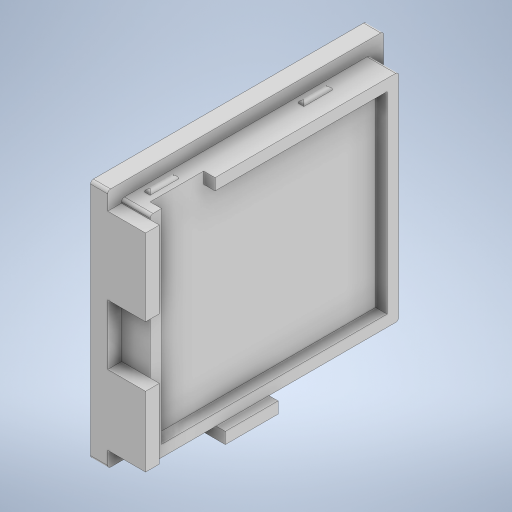
# Autodesk Inventor part: Enclosure_Bottom
Saved by Autodesk Inventor 2023 (Build 270158030, 158C)
## iProperties
Created: 2023-07-27
Part Number: Enclosure_Bottom
Material: Generic
Document SubType Name: Modeling
Designer: Tropaion
Density: 1 g/cm^3
Appearance: Default
Author: Tropaion
Autodesk Inventor part; units mm, degrees
ref_plane "YZ Plane" through (0, 0, 0) normal (1, 0, 0) x (0, 1, 0)
ref_plane "XZ Plane" through (0, 0, 0) normal (0, 1, 0) x (-1, 0, 0)
ref_plane "XY Plane" through (0, 0, 0) normal (0, 0, 1) x (1, 0, 0)
sketch "Sketch1" plane through (0, 0, 0) normal (1, 0, 0) x (0, 1, 0)
  line L0 (9.8886, 10.374) -> (-32.1114, 10.374)
  line L1 (-32.1114, 10.374) -> (-32.1114, -37.736)
  line L2 (-32.1114, -37.736) -> (9.8886, -37.736)
  line L3 (9.8886, -37.736) -> (9.8886, 10.374)
  point P0 (0, 0)
  dimension "d0" = 42
  dimension "d1" = 48.11
  constraints: 8 end point, 2 parallel, 1 horizontal, 1 perpendicular
  measures "d0" distance of L2.end L1.end
  measures "d1" distance of L1.end L0.end
extrude "Extrusion1" add sketch "Sketch1" along normal blind 3
sketch "Sketch2" plane through (3, 0, 0) normal (1, 0, 0) x (0, 0, -1)
  line L0 (-7.974, 7.4886) -> (35.336, 7.4886)
  line L1 (35.336, 7.4886) -> (35.336, -30.1114)
  line L2 (35.336, -30.1114) -> (-7.974, -30.1114)
  line L3 (-7.974, -30.1114) -> (-7.974, 7.4886)
  line L4 (37.736, 9.8886) -> (-10.374, 9.8886) projected
  line L5 (-10.374, 9.8886) -> (-10.374, -32.1114) projected
  line L6 (-10.374, -32.1114) -> (37.736, -32.1114) projected
  point P0 (0, 0)
  dimension "d4" = 43.31
  dimension "d6" = 2.4
  dimension "d7" = 2.4
  dimension "d20" = 2
  constraints: 8 end point, 2 parallel, 1 horizontal, 1 perpendicular
  measures "d4" distance of L1.end L2.end
  measures "d6" distance between parallel lines of L4 L0
  measures "d7" distance between parallel lines of L5 L3
  measures "d20" distance between parallel lines of L6 L2
extrude "Extrusion2" add sketch "Sketch2" along normal blind 3
fillet "Fillet1" radius 0.5 4 edges at (1.5, 9.8886, 10.374) (1.5, 9.8886, -37.736) (1.5, -32.1114, 10.374) (1.5, -32.1114, -37.736)
sketch "Sketch3" plane through (3, 0, 0) normal (1, 0, 0) x (0, 0, -1)
  line L0 (-10.374, 9.3886) -> (-10.374, -31.6114) projected
  line L1 (-7.974, -30.1114) -> (-7.974, 7.4886) projected
  line L2 (-10.374, -29.3114) -> (-7.974, -29.3114)
  line L3 (-7.974, -29.3114) -> (-7.974, -17.1114)
  line L4 (-7.974, -17.1114) -> (-10.374, -17.1114)
  line L5 (-10.374, -17.1114) -> (-10.374, -29.3114)
  line L6 (-9.874, -32.1114) -> (37.236, -32.1114) projected
  point P0 (0, 0)
  point P1 (-7.974, -29.6114)
  point P2 (-7.974, 6.9886)
  point P3 (-7.974, -29.3114)
  dimension "d12" = 12.2
  dimension "d13" = 2.8
  constraints: 8 end point, 2 parallel, 2 point on line, 1 horizontal, 1 perpendicular
  measures "d12" distance of L3.end L2.end
  measures "d13" distance between parallel lines of L2 L6
extrude "PowerSocket" add sketch "Sketch3" along normal blind 6.6
sketch "Sketch5" plane through (3, 0, 0) normal (1, 0, 0) x (0, 0, -1)
  line L0 (-10.374, 9.3886) -> (-10.374, -17.1114) projected
  line L1 (-7.974, -17.1114) -> (-7.974, 7.4886) projected
  line L2 (-10.374, -6.6114) -> (-7.974, -6.6114)
  line L3 (-7.974, -6.6114) -> (-7.974, 6.7886)
  line L4 (-7.974, 6.7886) -> (-10.374, 6.7886)
  line L5 (-10.374, 6.7886) -> (-10.374, -6.6114)
  line L6 (-7.974, -17.1114) -> (-10.374, -17.1114) projected
  line L7 (35.336, 7.4886) -> (-7.974, 7.4886) projected
  line L8 (37.236, 9.8886) -> (-9.874, 9.8886) projected
  point P0 (0, 0)
  point P1 (-10.374, 6.7886)
  point P2 (-7.974, -6.6114)
  dimension "d21" = 13.4
  dimension "d75" = 3.1
  constraints: 8 end point, 2 parallel, 2 point on line, 1 horizontal, 1 perpendicular
  measures "d21" distance of L3.end L2.end
  measures "d75" distance between parallel lines of L4 L8
extrude "RJ-12" add sketch "Sketch5" along normal blind 6.6 contours L4 L1 L2 L0
sketch "Sketch6" plane through (3, 0, 0) normal (1, 0, 0) x (0, 0, -1)
  line L0 (-9.874, -32.1114) -> (37.236, -32.1114) projected
  line L1 (-7.974, -30.1114) -> (35.336, -30.1114) projected
  line L2 (12.726, -32.1114) -> (3.526, -32.1114)
  line L3 (3.526, -32.1114) -> (3.526, -30.1114)
  line L4 (3.526, -30.1114) -> (12.726, -30.1114)
  line L5 (12.726, -30.1114) -> (12.726, -32.1114)
  line L6 (-10.374, -29.3114) -> (-10.374, -31.6114) projected
  point P0 (0, 0)
  dimension "d25" = 9.2
  dimension "d26" = 13.9
  constraints: 8 end point, 2 parallel, 2 point on line, 1 horizontal, 1 perpendicular
  measures "d25" distance of L3.end L4.end
  measures "d26" distance between parallel lines of L6 L3
extrude "USB-C" add sketch "Sketch6" along normal blind 6.6
sketch "Sketch7" plane through (6, 0, 0) normal (1, 0, 0) x (0, 0, -1)
  line L0 (35.336, 7.4886) -> (-7.974, 7.4886) projected
  line L1 (-7.974, 7.4886) -> (-5.974, 7.4886)
  line L2 (-5.974, 7.4886) -> (-5.974, -30.1114)
  line L3 (-7.974, -30.1114) -> (3.526, -30.1114) projected
  line L4 (-5.974, -30.1114) -> (-7.974, -30.1114)
  line L5 (-10.374, -29.3114) -> (-10.374, -31.6114) projected
  line L6 (-7.974, 7.4886) -> (-7.974, -17.1114) projected
  line L7 (-7.974, -30.1114) -> (-7.974, 7.4886)
  line L8 (35.336, -30.1114) -> (12.726, -30.1114) projected
  line L9 (-5.974, -30.1114) -> (35.336, -30.1114)
  line L10 (35.336, -30.1114) -> (35.336, -28.1114)
  line L11 (35.336, 7.4886) -> (35.336, -30.1114) projected
  line L12 (35.336, -28.1114) -> (-5.974, -28.1114)
  line L13 (35.336, -28.1114) -> (35.336, 7.4886)
  line L14 (35.336, 7.4886) -> (33.336, 7.4886)
  line L15 (33.336, 7.4886) -> (33.336, -28.1114)
  line L16 (33.336, 7.4886) -> (3.336, 7.4886)
  line L17 (3.336, 7.4886) -> (3.336, 5.4886)
  line L18 (3.336, 5.4886) -> (33.336, 5.4886)
  point P0 (0, 0)
  point P1 (-7.974, 6.7886)
  point P2 (-7.974, 6.6886)
  dimension "d29" = 2
  dimension "d30" = 2
  dimension "d31" = 2
  dimension "d32" = 2
  dimension "d33" = 30
  dimension "d34" = 2
  constraints: 26 end point, 8 point on line, 7 perpendicular, 1 collinear
  measures "d29" distance of L0.end L1.end
  measures "d30" distance of L2.end L4.end
  measures "d31" distance of L8.start L10.end
  measures "d32" distance of L0.start L14.end
  measures "d33" distance of L14.end L16.end
  measures "d34" distance of L16.end L17.end
extrude "Extrusion7" add sketch "Sketch7" along normal blind 2 contours L11 L12 L15 L0 | L15 L18 L17 L0 | L10 L8 L9 L3 L2 L12 | L2 L3 L7 L6 L0
sketch "Sketch8" plane through (3, -30.1114, -3.526) normal (0, -1, 0) x (1, 0, 0)
  line L0 (2, 8.5) -> (1, 8.5)
  line L1 (1, 8.5) -> (1, 3.5)
  line L2 (1, 3.5) -> (2, 3.5)
  line L3 (2, 3.5) -> (2, 8.5)
  line L4 (0, 11.5) -> (5, 11.5) projected
  line L5 (5, 11.5) -> (5, 0) projected
  line L6 (0, 13.4) -> (0, 0) projected
  point P0 (-3, 3.526)
  point P1 (2, 6)
  dimension "d37" = 1
  dimension "d38" = 5
  dimension "d39" = 5.5
  dimension "d60" = 1
  constraints: 8 end point, 2 parallel, 1 horizontal, 1 midpoint, 1 perpendicular
  measures "d37" distance of L2.end L1.end
  measures "d38" distance of L1.end L0.end
  measures "d39" distance from line of L4 point (2, 6)
  measures "d60" distance between parallel lines of L6 L1
extrude "Extrusion8" add sketch "Sketch8" along normal blind 0.5
fillet "Fillet3" radius 0.5 4 edges at (5, -30.6114, 2.474) (4, -30.6114, 2.474) (4.5, -30.6114, 4.974) (4.5, -30.6114, -0.026)
sketch "Sketch9" plane through (3, -30.1114, -35.336) normal (0, -1, 0) x (1, 0, 0)
  line L0 (2, 13.5) -> (1, 13.5)
  line L1 (1, 13.5) -> (1, 8.5)
  line L2 (1, 8.5) -> (2, 8.5)
  line L3 (2, 8.5) -> (2, 13.5)
  line L4 (5, 22.61) -> (5, 0) projected
  line L5 (0, 0) -> (5, 0) projected
  line L6 (0, 22.61) -> (0, -1.9) projected
  point P0 (-3, 35.336)
  point P1 (2, 11)
  dimension "d44" = 1
  dimension "d45" = 5
  dimension "d47" = 11
  dimension "d59" = 1
  constraints: 8 end point, 2 parallel, 1 horizontal, 1 midpoint, 1 perpendicular
  measures "d44" distance of L2.end L1.end
  measures "d45" distance of L1.end L0.end
  measures "d47" distance from line of L5 point (2, 11)
  measures "d59" distance between parallel lines of L6 L1
extrude "Extrusion9" add sketch "Sketch9" along normal blind 0.5
fillet "Fillet4" radius 0.5 4 edges at (5, -30.6114, -24.336) (4, -30.6114, -24.336) (4.5, -30.6114, -21.836) (4.5, -30.6114, -26.836)
sketch "Sketch10" plane through (3, 7.4886, 7.974) normal (0, 1, 0) x (1, 0, 0)
  line L0 (2, 34.81) -> (1, 34.81)
  line L1 (1, 34.81) -> (1, 29.81)
  line L2 (1, 29.81) -> (2, 29.81)
  line L3 (2, 29.81) -> (2, 34.81)
  line L4 (5, 43.31) -> (5, 11.31) projected
  line L5 (0, 43.31) -> (5, 43.31) projected
  line L6 (0, 45.21) -> (0, -1.9) projected
  point P0 (-3, 7.974)
  point P1 (2, 32.31)
  dimension "d51" = 1
  dimension "d52" = 5
  dimension "d54" = 11
  dimension "d58" = 1
  constraints: 8 end point, 2 parallel, 1 horizontal, 1 midpoint, 1 perpendicular
  measures "d51" distance of L2.end L1.end
  measures "d52" distance of L1.end L0.end
  measures "d54" distance from line of L5 point (2, 32.31)
  measures "d58" distance between parallel lines of L6 L1
extrude "Extrusion10" add sketch "Sketch10" along normal blind 0.5
fillet "Fillet5" radius 0.5 4 edges at (5, 7.9886, -24.336) (4, 7.9886, -24.336) (4.5, 7.9886, -26.836) (4.5, 7.9886, -21.836)
sketch "Sketch11" plane through (3, 7.4886, 7.974) normal (0, 1, 0) x (1, 0, 0)
  line L0 (2, 8) -> (1, 8)
  line L1 (1, 8) -> (1, 3)
  line L2 (1, 3) -> (2, 3)
  line L3 (2, 3) -> (2, 8)
  line L4 (0, 45.21) -> (0, -1.9) projected
  line L5 (0, 0) -> (5, 0) projected
  point P0 (-3, 7.974)
  point P1 (1, 5.5)
  dimension "d61" = 1
  dimension "d62" = 5
  dimension "d63" = 1
  dimension "d64" = 5.5
  constraints: 8 end point, 2 parallel, 1 horizontal, 1 midpoint, 1 perpendicular
  measures "d61" distance of L2.end L1.end
  measures "d62" distance of L1.end L0.end
  measures "d63" distance between parallel lines of L4 L1
  measures "d64" distance from line of point (1, 5.5) L5
extrude "Extrusion11" add sketch "Sketch11" along normal blind 0.5
fillet "Fillet6" radius 0.5 4 edges at (5, 7.9886, 2.474) (4, 7.9886, 2.474) (4.5, 7.9886, 4.974) (4.5, 7.9886, -0.026)
fillet "Fillet7" radius 0.5 4 edges at (5.5, -30.1114, -35.336) (5.5, 7.4886, -35.336) (5.5, 7.4886, 7.974) (5.5, -30.1114, 7.974)
body "Solid1"
